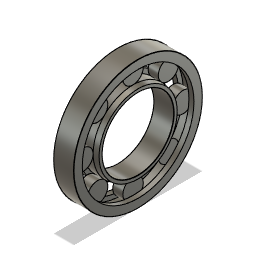
Bearing_GOST_8328-75_42000 (Autodesk Fusion 360 design; units mm, degrees)
Autodesk Fusion 360 part; units mm, degrees
sketch "Sketch1" plane through (0, 0, 0) normal (0, 0, 1) x (1, 0, 0)
  line L0 (-56.5, 0) -> (48.5, 0)
  line L1 (-42.5, 150) -> (-42.5, 186)
  line L2 (-42.5, 186) -> (-21.25, 186)
  line L3 (-21.25, 186) -> (-21.25, 167.4)
  line L4 (-21.25, 167.4) -> (21.25, 167.4)
  line L5 (21.25, 167.4) -> (42.5, 163.6531)
  line L6 (42.5, 163.6531) -> (42.5, 150)
  line L7 (42.5, 150) -> (-42.5, 150)
  line L8 (-42.5, 234) -> (-21.25, 234)
  line L9 (-21.25, 234) -> (-21.25, 252.6)
  line L10 (-21.25, 252.6) -> (21.25, 252.6)
  line L11 (21.25, 252.6) -> (21.25, 234)
  line L12 (21.25, 234) -> (42.5, 234)
  line L13 (42.5, 234) -> (42.5, 270)
  line L14 (42.5, 270) -> (-42.5, 270)
  line L15 (-42.5, 270) -> (-42.5, 234)
  line L16 (-21.25, 234) -> (-21.25, 186)
  line L17 (21.25, 234) -> (21.25, 167.4)
  line L18 (0, 252.6) -> (0, 167.4) construction
  line L19 (-21.25, 210) -> (21.25, 210)
  point P0 (0, 150)
  point P1 (0, 167.4)
  point P2 (0, 210)
  dimension "d1" = 300
  dimension "d2" = 10
  dimension "d3" = 85
  dimension "d4" = 21.25
  dimension "d6" = 540
  dimension "d7" = 505.2
  dimension "d9" = 468
  dimension "d10" = 372
  dimension "d20" = 334.8
  constraint horizontal L0
  constraint coincident L0 origin
  constraint vertical L1
  constraint perpendicular L1 L2
  constraint perpendicular L2 L3
  constraint perpendicular L1 L4
  constraint perpendicular L4 L6
  constraint perpendicular L6 L7
  constraint coincident L1.start L7.end
  constraint midpoint L7 P0
  constraint vertical origin P0
  constraint midpoint L4 P1
  constraint vertical P0 P1
  constraint horizontal L8
  constraint perpendicular L8 L9
  constraint perpendicular L9 L10
  constraint perpendicular L10 L11
  constraint perpendicular L11 L12
  constraint perpendicular L12 L13
  constraint perpendicular L11 L14
  constraint perpendicular L14 L15
  constraint vertical L2.end L8.end
  constraint vertical L1.end L8.start
  constraint vertical L4.end L11.end
  constraint vertical L5.end L12.end
  constraint horizontal L8.end L11.end
  constraint parallel L11 L17
  constraint midpoint L10 L18.start
  constraint coincident P1 L18.end
  constraint coincident L16 L19.start
  constraint coincident L17 L19.end
  constraint perpendicular L17 L19
  constraint midpoint L18 P2
  constraint coincident L19 P2
  measures "d2" angle of L4 L5
  measures "d3" distance of L1 L6
  measures "d4" horizontal distance of L4.end L5.end
revolve "Revolve1" add sketch "Sketch1" angle 360 about axis through (-56.5, 0, 0) along (1, 0, 0) contours L1 L2 L3 L4 L5 L6 L7 | L8 L9 L10 L11 L12 L13 L14 L15 makes body 1 at (14.1667, 269.6644, -13.4584) makes body 2 at (-14.1667, 149.2546, -14.9352)
revolve "Revolve2" add sketch "Sketch1" angle 360 about axis through (-21.25, 210, 0) along (1, 0, 0) separate body contours L9 L10 L11 L16 L17 L19 makes body 3
pattern_circular "C-Pattern1" count 8 over 360 about axis through (-56.5, 0, 0) along (1, 0, 0) of bodies 3 makes body 4 at (-7.0833, 180.0792, 177.0762) makes body 5 at (-7.0833, 2.1234, 252.547) makes body 6 at (-7.0833, -177.0762, 180.0792) makes body 7 at (-7.0833, -252.547, 2.1234) makes body 8 at (-7.0833, -180.0792, -177.0762) makes body 9 at (-7.0833, -2.1234, -252.547) makes body 10 at (-7.0833, 177.0762, -180.0792)
fillet "Fillet1" radius 1 2 edges at (42.5, -97.6362, 251.7284) (-42.5, -97.6362, 251.7284) on bodies 1
fillet "Fillet2" radius 1 2 edges at (42.5, -54.2423, 139.8491) (-42.5, -54.2423, 139.8491) on bodies 2
